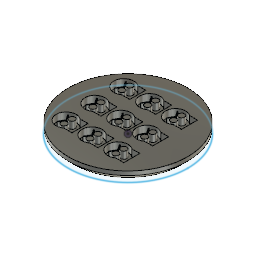
Semana3_Desafio5 v1 (Autodesk Fusion 360 design; units mm, degrees)
Autodesk Fusion 360 part; units mm, degrees
sketch "Sketch1" plane through (0, 0, 0) normal (0, 0, 1) x (1, 0, 0)
  circle A0 centre (0, 0) radius 30
  constraint coincident A0.centre origin
extrude "Extrude1" add sketch "Sketch1" along normal blind 5
sketch "Sketch2" plane through (0, 0, 5) normal (0, 0, 1) x (-1, 0, 0)
  circle A0 centre (0, 0) radius 30
  circle A1 centre (16.4954, -14.399) radius 5
  line L0 (13.4954, -10.399) -> (9.4954, -10.399)
  line L1 (9.4954, -10.399) -> (9.4954, -18.399)
  line L2 (9.4954, -18.399) -> (13.4954, -18.399)
  line L3 (12.4954, -11.399) -> (9.4954, -11.399)
  line L4 (9.4954, -12.399) -> (11.9128, -12.399)
  line L5 (9.4954, -13.399) -> (11.5964, -13.399)
  line L6 (9.4954, -14.399) -> (11.4954, -14.399)
  line L7 (9.4954, -15.399) -> (11.5964, -15.399)
  line L8 (9.4954, -16.399) -> (11.9128, -16.399)
  line L9 (9.4954, -17.399) -> (12.4954, -17.399)
  circle A2 centre (15.4954, -12.399) radius 1.5
  circle A3 centre (15.4954, -16.399) radius 1.5
  line L10 (16.4954, -13.899) -> (17.9954, -11.399)
  line L11 (17.9954, -11.399) -> (18.3005, -11.582)
  line L12 (18.3005, -11.582) -> (16.8356, -14.0235)
  line L13 (16.8356, -14.0235) -> (16.4954, -13.899)
  line L14 (18.4212, -17.1033) -> (18.1264, -17.3024)
  line L15 (16.5327, -14.9429) -> (16.7893, -14.6873)
  line L16 (18.1264, -17.3024) -> (16.5327, -14.9429)
  line L17 (16.7893, -14.6873) -> (18.4212, -17.1033)
  circle A4 centre (3.4954, -14.399) radius 5
  line L18 (-3.5046, -17.399) -> (-0.5046, -17.399)
  circle A5 centre (2.4954, -12.399) radius 1.5
  line L19 (-3.5046, -14.399) -> (-1.5046, -14.399)
  line L20 (-3.5046, -15.399) -> (-1.4036, -15.399)
  line L21 (0.4954, -10.399) -> (-3.5046, -10.399)
  line L22 (-3.5046, -13.399) -> (-1.4036, -13.399)
  circle A6 centre (2.4954, -16.399) radius 1.5
  line L23 (3.5327, -14.9429) -> (3.7893, -14.6873)
  line L24 (4.9954, -11.399) -> (5.3005, -11.582)
  line L25 (3.7893, -14.6873) -> (5.4212, -17.1033)
  line L26 (5.3005, -11.582) -> (3.8356, -14.0235)
  line L27 (-0.5046, -11.399) -> (-3.5046, -11.399)
  line L28 (-3.5046, -10.399) -> (-3.5046, -18.399)
  line L29 (-3.5046, -16.399) -> (-1.0872, -16.399)
  line L30 (3.8356, -14.0235) -> (3.4954, -13.899)
  line L31 (3.4954, -13.899) -> (4.9954, -11.399)
  line L32 (5.4212, -17.1033) -> (5.1264, -17.3024)
  line L33 (5.1264, -17.3024) -> (3.5327, -14.9429)
  line L34 (-3.5046, -12.399) -> (-1.0872, -12.399)
  line L35 (-3.5046, -18.399) -> (0.4954, -18.399)
  circle A7 centre (-9.5046, -14.399) radius 5
  line L36 (-16.5046, -17.399) -> (-13.5046, -17.399)
  circle A8 centre (-10.5046, -12.399) radius 1.5
  line L37 (-16.5046, -14.399) -> (-14.5046, -14.399)
  line L38 (-16.5046, -15.399) -> (-14.4036, -15.399)
  line L39 (-12.5046, -10.399) -> (-16.5046, -10.399)
  line L40 (-16.5046, -13.399) -> (-14.4036, -13.399)
  circle A9 centre (-10.5046, -16.399) radius 1.5
  line L41 (-9.4673, -14.9429) -> (-9.2107, -14.6873)
  line L42 (-8.0046, -11.399) -> (-7.6995, -11.582)
  line L43 (-9.2107, -14.6873) -> (-7.5788, -17.1033)
  line L44 (-7.6995, -11.582) -> (-9.1644, -14.0235)
  line L45 (-13.5046, -11.399) -> (-16.5046, -11.399)
  line L46 (-16.5046, -10.399) -> (-16.5046, -18.399)
  line L47 (-16.5046, -16.399) -> (-14.0872, -16.399)
  line L48 (-9.1644, -14.0235) -> (-9.5046, -13.899)
  line L49 (-9.5046, -13.899) -> (-8.0046, -11.399)
  line L50 (-7.5788, -17.1033) -> (-7.8736, -17.3024)
  line L51 (-7.8736, -17.3024) -> (-9.4673, -14.9429)
  line L52 (-16.5046, -12.399) -> (-14.0872, -12.399)
  line L53 (-16.5046, -18.399) -> (-12.5046, -18.399)
  circle A10 centre (16.4954, 0.101) radius 5
  line L54 (9.4954, -2.899) -> (12.4954, -2.899)
  circle A11 centre (15.4954, 2.101) radius 1.5
  line L55 (9.4954, 0.101) -> (11.4954, 0.101)
  line L56 (9.4954, -0.899) -> (11.5964, -0.899)
  line L57 (13.4954, 4.101) -> (9.4954, 4.101)
  line L58 (9.4954, 1.101) -> (11.5964, 1.101)
  circle A12 centre (15.4954, -1.899) radius 1.5
  line L59 (16.5327, -0.4429) -> (16.7893, -0.1873)
  line L60 (17.9954, 3.101) -> (18.3005, 2.918)
  line L61 (16.7893, -0.1873) -> (18.4212, -2.6033)
  line L62 (18.3005, 2.918) -> (16.8356, 0.4765)
  line L63 (12.4954, 3.101) -> (9.4954, 3.101)
  line L64 (9.4954, 4.101) -> (9.4954, -3.899)
  line L65 (9.4954, -1.899) -> (11.9128, -1.899)
  line L66 (16.8356, 0.4765) -> (16.4954, 0.601)
  line L67 (16.4954, 0.601) -> (17.9954, 3.101)
  line L68 (18.4212, -2.6033) -> (18.1264, -2.8024)
  line L69 (18.1264, -2.8024) -> (16.5327, -0.4429)
  line L70 (9.4954, 2.101) -> (11.9128, 2.101)
  line L71 (9.4954, -3.899) -> (13.4954, -3.899)
  circle A13 centre (3.4954, 0.101) radius 5
  line L72 (-3.5046, -2.899) -> (-0.5046, -2.899)
  circle A14 centre (2.4954, 2.101) radius 1.5
  line L73 (-3.5046, 0.101) -> (-1.5046, 0.101)
  line L74 (-3.5046, -0.899) -> (-1.4036, -0.899)
  line L75 (0.4954, 4.101) -> (-3.5046, 4.101)
  line L76 (-3.5046, 1.101) -> (-1.4036, 1.101)
  circle A15 centre (2.4954, -1.899) radius 1.5
  line L77 (3.5327, -0.4429) -> (3.7893, -0.1873)
  line L78 (4.9954, 3.101) -> (5.3005, 2.918)
  line L79 (3.7893, -0.1873) -> (5.4212, -2.6033)
  line L80 (5.3005, 2.918) -> (3.8356, 0.4765)
  line L81 (-0.5046, 3.101) -> (-3.5046, 3.101)
  line L82 (-3.5046, 4.101) -> (-3.5046, -3.899)
  line L83 (-3.5046, -1.899) -> (-1.0872, -1.899)
  line L84 (3.8356, 0.4765) -> (3.4954, 0.601)
  line L85 (3.4954, 0.601) -> (4.9954, 3.101)
  line L86 (5.4212, -2.6033) -> (5.1264, -2.8024)
  line L87 (5.1264, -2.8024) -> (3.5327, -0.4429)
  line L88 (-3.5046, 2.101) -> (-1.0872, 2.101)
  line L89 (-3.5046, -3.899) -> (0.4954, -3.899)
  circle A16 centre (-9.5046, 0.101) radius 5
  line L90 (-16.5046, -2.899) -> (-13.5046, -2.899)
  circle A17 centre (-10.5046, 2.101) radius 1.5
  line L91 (-16.5046, 0.101) -> (-14.5046, 0.101)
  line L92 (-16.5046, -0.899) -> (-14.4036, -0.899)
  line L93 (-12.5046, 4.101) -> (-16.5046, 4.101)
  line L94 (-16.5046, 1.101) -> (-14.4036, 1.101)
  circle A18 centre (-10.5046, -1.899) radius 1.5
  line L95 (-9.4673, -0.4429) -> (-9.2107, -0.1873)
  line L96 (-8.0046, 3.101) -> (-7.6995, 2.918)
  line L97 (-9.2107, -0.1873) -> (-7.5788, -2.6033)
  line L98 (-7.6995, 2.918) -> (-9.1644, 0.4765)
  line L99 (-13.5046, 3.101) -> (-16.5046, 3.101)
  line L100 (-16.5046, 4.101) -> (-16.5046, -3.899)
  line L101 (-16.5046, -1.899) -> (-14.0872, -1.899)
  line L102 (-9.1644, 0.4765) -> (-9.5046, 0.601)
  line L103 (-9.5046, 0.601) -> (-8.0046, 3.101)
  line L104 (-7.5788, -2.6033) -> (-7.8736, -2.8024)
  line L105 (-7.8736, -2.8024) -> (-9.4673, -0.4429)
  line L106 (-16.5046, 2.101) -> (-14.0872, 2.101)
  line L107 (-16.5046, -3.899) -> (-12.5046, -3.899)
  circle A19 centre (16.4954, 14.601) radius 5
  line L108 (9.4954, 11.601) -> (12.4954, 11.601)
  circle A20 centre (15.4954, 16.601) radius 1.5
  line L109 (9.4954, 14.601) -> (11.4954, 14.601)
  line L110 (9.4954, 13.601) -> (11.5964, 13.601)
  line L111 (13.4954, 18.601) -> (9.4954, 18.601)
  line L112 (9.4954, 15.601) -> (11.5964, 15.601)
  circle A21 centre (15.4954, 12.601) radius 1.5
  line L113 (16.5327, 14.0571) -> (16.7893, 14.3127)
  line L114 (17.9954, 17.601) -> (18.3005, 17.418)
  line L115 (16.7893, 14.3127) -> (18.4212, 11.8967)
  line L116 (18.3005, 17.418) -> (16.8356, 14.9765)
  line L117 (12.4954, 17.601) -> (9.4954, 17.601)
  line L118 (9.4954, 18.601) -> (9.4954, 10.601)
  line L119 (9.4954, 12.601) -> (11.9128, 12.601)
  line L120 (16.8356, 14.9765) -> (16.4954, 15.101)
  line L121 (16.4954, 15.101) -> (17.9954, 17.601)
  line L122 (18.4212, 11.8967) -> (18.1264, 11.6976)
  line L123 (18.1264, 11.6976) -> (16.5327, 14.0571)
  line L124 (9.4954, 16.601) -> (11.9128, 16.601)
  line L125 (9.4954, 10.601) -> (13.4954, 10.601)
  circle A22 centre (3.4954, 14.601) radius 5
  line L126 (-3.5046, 11.601) -> (-0.5046, 11.601)
  circle A23 centre (2.4954, 16.601) radius 1.5
  line L127 (-3.5046, 14.601) -> (-1.5046, 14.601)
  line L128 (-3.5046, 13.601) -> (-1.4036, 13.601)
  line L129 (0.4954, 18.601) -> (-3.5046, 18.601)
  line L130 (-3.5046, 15.601) -> (-1.4036, 15.601)
  circle A24 centre (2.4954, 12.601) radius 1.5
  line L131 (3.5327, 14.0571) -> (3.7893, 14.3127)
  line L132 (4.9954, 17.601) -> (5.3005, 17.418)
  line L133 (3.7893, 14.3127) -> (5.4212, 11.8967)
  line L134 (5.3005, 17.418) -> (3.8356, 14.9765)
  line L135 (-0.5046, 17.601) -> (-3.5046, 17.601)
  line L136 (-3.5046, 18.601) -> (-3.5046, 10.601)
  line L137 (-3.5046, 12.601) -> (-1.0872, 12.601)
  line L138 (3.8356, 14.9765) -> (3.4954, 15.101)
  line L139 (3.4954, 15.101) -> (4.9954, 17.601)
  line L140 (5.4212, 11.8967) -> (5.1264, 11.6976)
  line L141 (5.1264, 11.6976) -> (3.5327, 14.0571)
  line L142 (-3.5046, 16.601) -> (-1.0872, 16.601)
  line L143 (-3.5046, 10.601) -> (0.4954, 10.601)
  circle A25 centre (-9.5046, 14.601) radius 5
  line L144 (-16.5046, 11.601) -> (-13.5046, 11.601)
  circle A26 centre (-10.5046, 16.601) radius 1.5
  line L145 (-16.5046, 14.601) -> (-14.5046, 14.601)
  line L146 (-16.5046, 13.601) -> (-14.4036, 13.601)
  line L147 (-12.5046, 18.601) -> (-16.5046, 18.601)
  line L148 (-16.5046, 15.601) -> (-14.4036, 15.601)
  circle A27 centre (-10.5046, 12.601) radius 1.5
  line L149 (-9.4673, 14.0571) -> (-9.2107, 14.3127)
  line L150 (-8.0046, 17.601) -> (-7.6995, 17.418)
  line L151 (-9.2107, 14.3127) -> (-7.5788, 11.8967)
  line L152 (-7.6995, 17.418) -> (-9.1644, 14.9765)
  line L153 (-13.5046, 17.601) -> (-16.5046, 17.601)
  line L154 (-16.5046, 18.601) -> (-16.5046, 10.601)
  line L155 (-16.5046, 12.601) -> (-14.0872, 12.601)
  line L156 (-9.1644, 14.9765) -> (-9.5046, 15.101)
  line L157 (-9.5046, 15.101) -> (-8.0046, 17.601)
  line L158 (-7.5788, 11.8967) -> (-7.8736, 11.6976)
  line L159 (-7.8736, 11.6976) -> (-9.4673, 14.0571)
  line L160 (-16.5046, 16.601) -> (-14.0872, 16.601)
  line L161 (-16.5046, 10.601) -> (-12.5046, 10.601)
  point P0 (16.3362, -14.476)
  point P1 (3.3362, -14.476)
  point P2 (-9.6638, -14.476)
  point P3 (16.3362, 0.024)
  point P4 (3.3362, 0.024)
  point P5 (-9.6638, 0.024)
  point P6 (16.3362, 14.524)
  point P7 (3.3362, 14.524)
  point P8 (-9.6638, 14.524)
  dimension "d5" = -26
  dimension "d6" = 29
  constraint coincident A1 L0.start
  constraint horizontal L0
  constraint perpendicular L0 L1
  constraint coincident A1 L2.end
  constraint perpendicular L1 L2
  constraint coincident A1 L3.start
  constraint coincident L1 L3.end
  constraint perpendicular L1 L3
  constraint coincident L1 L4.start
  constraint coincident A1 L4.end
  constraint perpendicular L1 L4
  constraint coincident L1 L5.start
  constraint coincident A1 L5.end
  constraint perpendicular L1 L5
  constraint midpoint L1 L6.start
  constraint coincident A1 L6.end
  constraint perpendicular L1 L6
  constraint coincident L1 L7.start
  constraint coincident A1 L7.end
  constraint perpendicular L1 L7
  constraint coincident L1 L8.start
  constraint coincident A1 L8.end
  constraint perpendicular L1 L8
  constraint coincident L1 L9.start
  constraint coincident A1 L9.end
  constraint perpendicular L1 L9
  constraint perpendicular L10 L11
  constraint perpendicular L11 L12
  constraint perpendicular L14 L17
  constraint perpendicular L14 L16
extrude "Extrude2" cut sketch "Sketch2" against normal blind 3.5 contours A1 | A1 L0 L1 L3 | A1 L1 L2 L9 | A1 L1 L3 L4 | A1 L1 L8 L9 | A1 L1 L4 L5 | A1 L1 L7 L8 | A1 L1 L5 L6 | A1 L1 L6 L7 | A2 | A3 | L10 L11 L12 L13 | L14 L15 L16 L17 | A4 | A4 L21 L27 L28 | A4 L18 L28 L35 | A4 L27 L28 L34 | A4 L18 L28 L29 | A4 L22 L28 L34 | A4 L20 L28 L29 | A4 L19 L22 L28 | A4 L19 L20 L28 | A5 | A6 | L23 L25 L32 L33 | L24 L26 L30 L31 | A7 | A7 L39 L45 L46 | A7 L36 L46 L53 | A7 L45 L46 L52 | A7 L36 L46 L47 | A7 L40 L46 L52 | A7 L38 L46 L47 | A7 L37 L40 L46 | A7 L37 L38 L46 | A8 | A9 | L41 L43 L50 L51 | L42 L44 L48 L49 | A10 | A10 L57 L63 L64 | A10 L54 L64 L71 | A10 L63 L64 L70 | A10 L54 L64 L65 | A10 L58 L64 L70 | A10 L56 L64 L65 | A10 L55 L58 L64 | A10 L55 L56 L64 | A11 | A12 | L59 L61 L68 L69 | L60 L62 L66 L67 | A13 | A13 L75 L81 L82 | A13 L72 L82 L89 | A13 L81 L82 L88 | A13 L72 L82 L83 | A13 L76 L82 L88 | A13 L74 L82 L83 | A13 L73 L76 L82 | A13 L73 L74 L82 | A14 | A15 | L77 L79 L86 L87 | L78 L80 L84 L85 | A16 | A16 L93 L99 L100 | A16 L90 L100 L107 | A16 L99 L100 L106 | A16 L90 L100 L101 | A16 L94 L100 L106 | A16 L92 L100 L101 | A16 L91 L94 L100 | A16 L91 L92 L100 | A17 | A18 | L95 L97 L104 L105 | L96 L98 L102 L103 | A19 | A19 L111 L117 L118 | A19 L108 L118 L125 | A19 L117 L118 L124 | A19 L108 L118 L119 | A19 L112 L118 L124 | A19 L110 L118 L119 | A19 L109 L112 L118 | A19 L109 L110 L118 | A20 | A21 | L113 L115 L122 L123 | L114 L116 L120 L121 | A22 | A22 L129 L135 L136 | A22 L126 L136 L143 | A22 L135 L136 L142 | A22 L126 L136 L137 | A22 L130 L136 L142 | A22 L128 L136 L137 | A22 L127 L130 L136 | A22 L127 L128 L136 | A23 | A24 | L131 L133 L140 L141 | L132 L134 L138 L139 | A25 | A25 L147 L153 L154 | A25 L144 L154 L161 | A25 L153 L154 L160 | A25 L144 L154 L155 | A25 L148 L154 L160 | A25 L146 L154 L155 | A25 L145 L148 L154 | A25 L145 L146 L154 | A26 | A27 | L149 L151 L158 L159 | L150 L152 L156 L157
extrude "Extrude3" add sketch "Sketch2" against normal blind 4 contours A2 | A3 | L10 L11 L12 L13 | L14 L15 L16 L17 | A5 | A6 | L23 L25 L32 L33 | L24 L26 L30 L31 | A8 | A9 | L41 L43 L50 L51 | L42 L44 L48 L49 | A11 | A12 | L59 L61 L68 L69 | L60 L62 L66 L67 | A14 | A15 | L77 L79 L86 L87 | L78 L80 L84 L85 | A17 | A18 | L95 L97 L104 L105 | L96 L98 L102 L103 | A20 | A21 | L113 L115 L122 L123 | L114 L116 L120 L121 | A23 | A24 | L131 L133 L140 L141 | L132 L134 L138 L139 | A26 | A27 | L149 L151 L158 L159 | L150 L152 L156 L157
chamfer "Chamfer1" distance 3 angle 45 1 edges at (-27.9698, -10.8485, 0)
